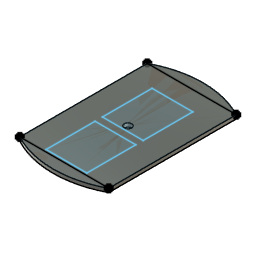
Phoenix 2eme plaque (Autodesk Fusion 360 design; units mm, degrees)
Autodesk Fusion 360 part; units mm, degrees
sketch "Esquisse1" plane through (0, 0, 0) normal (0, 0, 1) x (1, 0, 0)
  line L0 (60, -86) -> (-60, -86)
  line L1 (-60, -86) -> (-60, 86)
  line L2 (-60, 86) -> (60, 86)
  line L3 (60, 86) -> (60, -86)
  line L4 (60, -86) -> (-60, 86) construction
  line L5 (-60, -86) -> (60, 86) construction
  dimension "d1" = 120
  dimension "d2" = 172
  constraint horizontal L0
  constraint perpendicular L0 L1
  constraint parallel L0 L2
  constraint parallel L1 L3
  constraint coincident L4 origin
  constraint coincident L5 origin
  measures "d1" distance of L1.end L2.end
  measures "d2" distance of L0.end L1.end
sketch "Esquisse2" plane through (0, 0, 0) normal (0, 0, 1) x (1, 0, 0)
  line L0 (0, -86) -> (0, -101)
  line L1 (0, 86) -> (0, 101)
  line L2 (60, -86) -> (-60, -86)
  line L3 (-60, -86) -> (-60, -116)
  line L4 (-60, -116) -> (60, -116)
  line L5 (60, -116) -> (60, -86)
  line L6 (60, -86) -> (-60, -116) construction
  line L7 (-60, -86) -> (60, -116) construction
  line L8 (-60, 86) -> (60, 86)
  line L9 (60, 86) -> (60, 116)
  line L10 (60, 116) -> (-60, 116)
  line L11 (-60, 116) -> (-60, 86)
  line L12 (-60, 86) -> (60, 116) construction
  line L13 (60, 86) -> (-60, 116) construction
  arc A0 (60, 86) -> (-60, 86) centre (0, -26.5) ccw
  arc A1 (-60, -86) -> (60, -86) centre (0, 26.5) ccw
  point P0 (0, -101)
  point P1 (0, 101)
  dimension "d3" = 15
  dimension "d4" = 15
  constraint vertical L0
  constraint vertical L1
  constraint horizontal L2
  constraint perpendicular L2 L3
  constraint parallel L2 L4
  constraint parallel L3 L5
  constraint coincident L6 P0
  constraint coincident L7 P0
  constraint coincident P0 L0.end
  constraint horizontal L8
  constraint perpendicular L8 L9
  constraint parallel L8 L10
  constraint parallel L9 L11
  constraint coincident L12 P1
  constraint coincident L13 P1
  constraint coincident P1 L1.end
  constraint coincident P1 A0
  constraint coincident P0 A1
  measures "d3" distance of L0.start P0
  measures "d4" distance of L1.start P1
extrude "Extrusion1" add sketch "Esquisse1" sketch "Esquisse2" along normal blind 10 of sketch 2 contours L0 L2 A1 | L0 L2 A1 | L1 L8 A0 | L1 L8 A0
sketch "Esquisse3" plane through (0, 0, 10) normal (0, 0, 1) x (-1, 0, 0)
  line L0 (60, -86) -> (60, 86)
  arc A0 (60, 86) -> (-60, 86) centre (0, -26.5) ccw
  line L1 (-60, 86) -> (-60, -86)
  arc A1 (-60, -86) -> (60, -86) centre (0, 26.5) ccw
  line L2 (60, 86) -> (-60, 86)
  line L3 (60, -86) -> (-60, -86)
  line L4 (-60, 86) -> (-60, 70)
  line L5 (-60, 70) -> (-60, 48)
  line L6 (-60, 48) -> (-60, -48)
  line L7 (-60, -48) -> (-60, -70)
  line L8 (60, 86) -> (60, 70)
  line L9 (60, 70) -> (60, 48)
  line L10 (60, 48) -> (60, -48)
  line L11 (60, -48) -> (60, -70)
  line L12 (60, 70) -> (36, 70)
  line L13 (36, 70) -> (36, 48)
  line L14 (36, 48) -> (60, 48)
  line L15 (60, -70) -> (36, -70)
  line L16 (36, -70) -> (36, -48)
  line L17 (36, -48) -> (60, -48)
  line L18 (-60, -70) -> (-36, -70)
  line L19 (-36, -70) -> (-36, -48)
  line L20 (-36, -48) -> (-60, -48)
  line L21 (-60, 70) -> (-36, 70)
  line L22 (-36, 70) -> (-36, 48)
  line L23 (-60, 48) -> (-36, 48)
  dimension "d7" = 16
  dimension "d8" = 22
  dimension "d9" = 96
  dimension "d10" = 22
  dimension "d11" = 16
  dimension "d12" = 22
  dimension "d13" = 96
  dimension "d14" = 22
  dimension "d15" = 24
  dimension "d16" = 24
  dimension "d17" = 22
  constraint coincident L0.end A0.start
  constraint coincident A0.end L1.start
  constraint coincident L0.start A1.end
  constraint coincident L1.end A1.start
  constraint perpendicular L2 L4
  constraint parallel L1 L5
  constraint parallel L1 L6
  constraint parallel L1 L7
  constraint perpendicular L2 L8
  constraint parallel L0 L9
  constraint parallel L0 L10
  constraint coincident L0 L11.end
  constraint perpendicular L0 L12
  constraint perpendicular L12 L13
  constraint perpendicular L9 L14
  constraint perpendicular L13 L15
  constraint perpendicular L15 L16
  constraint parallel L15 L17
  constraint perpendicular L7 L18
  constraint perpendicular L18 L19
  constraint horizontal L20
  constraint perpendicular L4 L21
  constraint perpendicular L21 L22
  constraint perpendicular L22 L23
  measures "d7" distance of A0.end L4.end
  measures "d8" distance of L4.end L5.end
  measures "d9" distance of L5.end L6.end
  measures "d10" distance of L6.end L7.end
  measures "d11" distance of L0.end L8.end
  measures "d12" distance of L8.end L9.end
  measures "d13" distance of L9.end L10.end
  measures "d14" distance of L10.end L11.end
  measures "d15" distance of L8.end L12.end
  measures "d16" distance of L7.end L18.end
  measures "d17" distance of L21.end L22.end
sketch "Esquisse4" plane through (0, 0, 10) normal (0, 0, 1) x (-1, 0, 0)
  line L0 (-60, -86) -> (-17, -86)
  line L1 (-17, -86) -> (17, -86)
  line L2 (17, -86) -> (17, -70)
  line L3 (17, -70) -> (-17, -70)
  line L4 (-17, -70) -> (-17, -86)
  dimension "d18" = 43
  dimension "d19" = 34
  constraint horizontal L0
  constraint horizontal L1
  constraint vertical L2
  constraint horizontal L3
  constraint vertical L4
  measures "d18" distance of L0.start L0.end
  measures "d19" distance of L0.end L1.end
extrude "Extrusion2" cut sketch "Esquisse3" against normal blind 5
extrude "Extrusion3" cut sketch "Esquisse4" along normal blind 0 and the other way blind 25
sketch "Esquisse5" plane through (0, 0, 5) normal (0, 0, 1) x (-1, 0, 0)
  line L0 (17, -86) -> (-17, -86)
  line L1 (-17, -86) -> (-17, -70)
  line L2 (-17, -70) -> (17, -70)
  line L3 (17, -70) -> (17, -86)
  arc A0 (60, 86) -> (-60, 86) centre (0, -26.5) ccw
  line L4 (-60, 86) -> (-60, -86)
  arc A1 (-60, -86) -> (60, -86) centre (0, 26.5) ccw
  line L5 (60, -86) -> (60, 86)
  line L6 (-60, -86) -> (60, -86)
  line L7 (-60, 86) -> (60, 86)
  line L8 (-60, -86) -> (-60, -70)
  line L9 (-60, -70) -> (-60, -48)
  line L10 (-60, -48) -> (-60, 48)
  line L11 (-60, 48) -> (-60, 70)
  line L12 (-60, -70) -> (-36, -70)
  line L13 (-36, -70) -> (-36, -48)
  line L14 (-36, -48) -> (-60, -48)
  line L15 (-60, 70) -> (-36, 70)
  line L16 (-60, 48) -> (-36, 48)
  line L17 (-36, 48) -> (-36, 70)
  line L18 (60, -70) -> (36, -70)
  line L19 (36, -70) -> (36, -48)
  line L20 (36, -48) -> (60, -48)
  line L21 (60, 48) -> (36, 48)
  line L22 (36, 48) -> (36, 70)
  line L23 (36, 70) -> (60, 70)
  dimension "d27" = 16
  dimension "d28" = 22
  dimension "d29" = 96
  dimension "d30" = 22
  dimension "d31" = 24
  dimension "d32" = 24
  constraint coincident L4.end A1.start
  constraint coincident A1.end L5.start
  constraint coincident A0.end L4.start
  constraint coincident A0.start L5.end
  constraint perpendicular L7 L8
  constraint coincident L4 L9.end
  constraint coincident L4 L10.end
  constraint parallel L4 L11
  constraint perpendicular L8 L12
  constraint perpendicular L12 L13
  constraint horizontal L14
  constraint perpendicular L13 L15
  constraint perpendicular L11 L16
  constraint vertical L17
  constraint coincident L5 L18.start
  constraint perpendicular L5 L18
  constraint perpendicular L14 L19
  constraint coincident L5 L20.end
  constraint perpendicular L13 L20
  constraint coincident L5 L21.start
  constraint perpendicular L5 L21
  constraint perpendicular L21 L22
  constraint coincident L5 L23.end
  constraint perpendicular L5 L23
  measures "d27" distance of L4.end L8.end
  measures "d28" distance of L8.end L9.end
  measures "d29" distance of L9.end L10.end
  measures "d30" distance of L10.end L11.end
  measures "d31" distance of L8.end L12.end
  measures "d32" distance of L18.start L18.end
sketch "Esquisse6" plane through (0, 0, 5) normal (0, 0, 1) x (-1, 0, 0)
  line L0 (27.5, -60) -> (-27.5, -60)
  line L1 (-27.5, -60) -> (-27.5, 7)
  line L2 (-27.5, 7) -> (27.5, 7)
  line L3 (27.5, 7) -> (27.5, -60)
  dimension "d34" = 55
  dimension "d35" = 67
  constraint horizontal L0
  constraint vertical L1
  constraint horizontal L2
  constraint vertical L3
  measures "d34" distance of L0.start L0.end
  measures "d35" distance of L0.start L2.end
sketch "Esquisse7" plane through (0, 0, 5) normal (0, 0, 1) x (-1, 0, 0)
  line L0 (27.5, 17) -> (-27.5, 17)
  line L1 (-27.5, 17) -> (-27.5, 83)
  line L2 (-27.5, 83) -> (27.5, 83)
  line L3 (27.5, 83) -> (27.5, 17)
  dimension "d38" = 55
  dimension "d39" = 66
  constraint horizontal L0
  constraint vertical L1
  constraint horizontal L2
  constraint vertical L3
  measures "d38" distance of L0.start L0.end
  measures "d39" distance of L0.start L2.end
extrude "Extrusion4" add sketch "Esquisse5" against normal blind 5 contours L0 L1 L2 L3 L6
sketch "Esquisse8" plane through (0, 0, 5) normal (0, 0, 1) x (-1, 0, 0)
  arc A0 (60, 86) -> (-60, 86) centre (0, -26.5) ccw
  line L0 (-60, 86) -> (-60, -86)
  arc A1 (-60, -86) -> (60, -86) centre (0, 26.5) ccw
  line L1 (60, -86) -> (60, 86)
  circle A2 centre (0, 0) radius 5
  dimension "d42" = 10
  constraint coincident A2.centre origin
  measures "d42" diameter of A2
extrude "Extrusion5" cut sketch "Esquisse8" against normal blind 5 contours A2
sketch "Esquisse9" plane through (0, 0, 5) normal (0, 0, 1) x (-1, 0, 0)
  circle A0 centre (0, 0) radius 5
  arc A1 (60, 86) -> (-60, 86) centre (0, -26.5) ccw
  line L0 (-60, 86) -> (-60, -86)
  arc A2 (-60, -86) -> (60, -86) centre (0, 26.5) ccw
  line L1 (60, -86) -> (60, 86)
  line L2 (60, 86) -> (-60, 86)
  line L3 (60, -86) -> (-60, -86)
  constraint coincident A1.start L1.end
  constraint coincident A1.end L0.start
  constraint coincident A2.end L1.start
  constraint coincident L0.end A2.start
